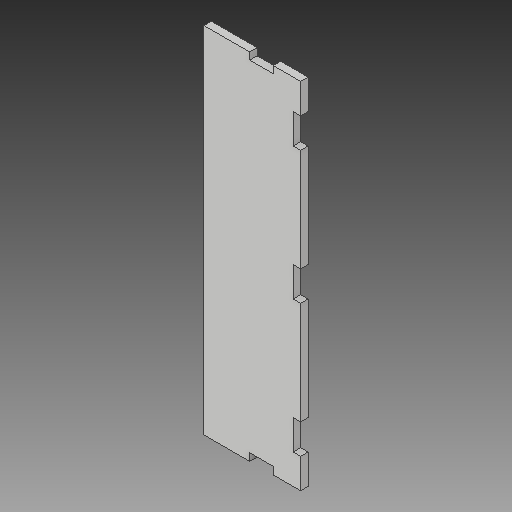
# Autodesk Inventor part: 1-8inch_Top2_1-Part
Saved by Autodesk Inventor 2018 (Build 220112000, 112)
## iProperties
Created: 2018-02-01
Part Number: 1-8inch_Top2_1-Part
Material: Generic
Document SubType Name: Modeling
Designer: Angie
Density: 1 g/cm^3
Appearance: Default
Author: Angie
Autodesk Inventor part; units mm, degrees
ref_plane "YZ Plane" through (0, 0, 0) normal (1, 0, 0) x (0, 1, 0)
ref_plane "XZ Plane" through (0, 0, 0) normal (0, 1, 0) x (-1, 0, 0)
ref_plane "XY Plane" through (0, 0, 0) normal (0, 0, 1) x (1, 0, 0)
sketch "Sketch1" plane through (0, 0, 0) normal (0, 0, 1) x (1, 0, 0)
  line L0 (-11.5, -148.5) -> (-11.5, -147.1375)
  line L1 (-21.5, -147.1375) -> (-21.5, -148.5)
  line L2 (-41, -148.5) -> (-41, 0.5)
  line L3 (-41, 0.5) -> (-21.5, 0.5)
  line L4 (-21.5, 0.5) -> (-21.5, -2.5)
  line L5 (-21.5, -2.5) -> (-11.5, -2.5)
  line L6 (-11.5, -2.5) -> (-11.5, 0.5)
  line L7 (-11.5, 0.5) -> (0, 0.5)
  line L8 (-11.5, -148.5) -> (-11.5, -147.1375)
  line L9 (-21.5, -147.1375) -> (-21.5, -148.5)
  line L10 (-41, -148.5) -> (-41, 0.5)
  line L11 (-41, 0.5) -> (-21.5, 0.5)
  line L12 (-21.5, 0.5) -> (-21.5, -2.5)
  line L13 (-21.5, -2.5) -> (-11.5, -2.5)
  line L14 (-11.5, -2.5) -> (-11.5, 0.5)
  line L15 (-11.5, 0.5) -> (0, 0.5)
  line L16 (-41, -150.3125) -> (-41, 0.5)
  line L17 (-11.5, -150.3125) -> (-11.5, -147.1375)
  line L18 (-11.5, -147.1375) -> (-21.5, -147.1375)
  line L19 (-21.5, -147.1375) -> (-21.5, -150.3125)
  line L20 (0, -150.3125) -> (-11.5, -150.3125)
  line L21 (-21.5, -150.3125) -> (-41, -150.3125)
  line L22 (0, 0.5) -> (-3.175, 0.5)
  line L23 (-3.175, -150.3125) -> (0, -150.3125)
  line L24 (-3.175, 0.5) -> (0, 0.5)
  line L25 (0, -12.2) -> (-2.9972, -12.2)
  line L26 (-2.9972, -12.2) -> (0, -12.2)
  line L27 (0, -24.9) -> (-2.9972, -24.9)
  line L28 (-2.9972, -24.9) -> (0, -24.9)
  line L29 (0, -68.5562) -> (-2.9972, -68.5562)
  line L30 (-2.9972, -68.5562) -> (0, -68.5562)
  line L31 (0, -81.2562) -> (-2.9972, -81.2562)
  line L32 (-2.9972, -81.2562) -> (0, -81.2562)
  line L33 (0, -124.9125) -> (-2.9972, -124.9125)
  line L34 (-2.9972, -124.9125) -> (0, -124.9125)
  line L35 (-3.175, -150.3125) -> (-0.1778, -150.3125)
  line L36 (-41, 0.5) -> (-21.5, 0.5)
  line L37 (-11.5, 0.5) -> (0, 0.5)
  line L38 (-2.9972, -12.2) -> (-2.9972, -24.9)
  line L39 (-2.9972, -68.5562) -> (-2.9972, -81.2562)
  line L40 (-2.9972, -124.9125) -> (-2.9972, -137.6125)
  line L41 (-0.1778, -150.3125) -> (0, -150.3125)
  line L42 (0, -124.9125) -> (0, -124.9125)
  line L43 (0, -81.2562) -> (0, -81.2562)
  line L44 (0, -68.5562) -> (0, -68.5562)
  line L45 (0, -24.9) -> (0, -24.9)
  line L46 (0, -12.2) -> (0, -12.2)
  line L47 (0, 0.5) -> (0, 0.5)
  line L48 (0, 0.5) -> (0.1778, 0.5)
  line L49 (0.1778, 0.5) -> (0.1778, -12.2)
  line L50 (0.1778, -12.2) -> (0, -12.2)
  line L51 (0, -24.9) -> (0.1778, -24.9)
  line L52 (0.1778, -24.9) -> (0.1778, -68.5562)
  line L53 (0.1778, -68.5562) -> (0, -68.5562)
  line L54 (0, -81.2562) -> (0.1778, -81.2562)
  line L55 (0.1778, -81.2562) -> (0.1778, -124.9125)
  line L56 (0.1778, -124.9125) -> (0, -124.9125)
  line L57 (-2.9972, -137.6125) -> (0.1778, -137.6125)
  line L58 (0.1778, -137.6125) -> (0.1778, -150.3125)
  line L59 (0.1778, -150.3125) -> (0, -150.3125)
  point P0 (0, 0)
  dimension "d0" = 150.8125
  dimension "d1" = 3.175
  dimension "d2" = 3.175
  dimension "d3" = 12.7
  dimension "d4" = 12.7
  dimension "d5" = 43.6562
  dimension "d6" = 12.7
  dimension "d7" = 43.6562
  dimension "d15" = 0.1778
  dimension "d18" = 0.1778
  constraints: 120 end point, 16 parallel, 15 horizontal, 6 perpendicular, 3 point on line
  measures "d0" distance of L22.start L20.start
  measures "d1" distance of L0.end L17.start
  measures "d2" distance of L23.end L23.start
  measures "d3" distance of L25.start L24.end
  measures "d4" distance of L25.start L27.start
  measures "d5" distance of L29.start L27.start
  measures "d6" distance of L29.start L31.start
  measures "d7" distance of L31.start L33.start
  measures "d15" distance of L23.end L35.end
  measures "d18" distance of L25.start L49.end
extrude "Extrusion3" add sketch "Sketch1" along normal blind 3.175
body "Solid3"
